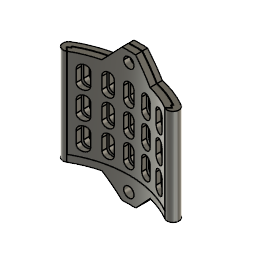
Mark 10 (Fusion) (Autodesk Fusion 360 design; units mm, degrees)
Autodesk Fusion 360 part; units mm, degrees
sketch "Base" plane through (0, 0, 0) normal (0, 0, 1) x (1, 0, 0) in component "Mark 10"
  circle A0 centre (0, 0) radius 57.15
  line L0 (0, 0) -> (0, 91.0821) construction
  line L1 (0, 0) -> (-28.575, 49.4934) construction
  line L2 (0, 0) -> (57.15, 0) construction
  circle A1 centre (-30.325, 52.5244) radius 3.5
  line L3 (-28.575, 49.4934) -> (-32.075, 55.5555) construction
  line L4 (-32.075, 55.5555) -> (-31.209, 56.0555) construction
  line L5 (-31.209, 56.0555) -> (-29.209, 52.5914)
  line L6 (-29.209, 52.5914) -> (-30.941, 51.5914)
  line L7 (-30.941, 51.5914) -> (-28.575, 49.4934)
  line L8 (0, 57.15) -> (0, 61.15) construction
  circle A2 centre (0, 0) radius 61.15
  line L9 (0, 57.15) -> (0, 64.15) construction
  circle A3 centre (0, 0) radius 64.15
  line L10 (28.575, 49.4934) -> (32.075, 55.5555) construction
  line L11 (32.075, 55.5555) -> (31.209, 56.0555) construction
  line L12 (31.209, 56.0555) -> (29.209, 52.5914)
  line L13 (30.941, 51.5914) -> (28.575, 49.4934)
  line L14 (29.209, 52.5914) -> (30.941, 51.5914)
  circle A4 centre (30.325, 52.5244) radius 3.5
  circle A5 centre (0, 0) radius 92.9081
  point P0 (-29.7049, 53.4504)
  point P1 (-29.209, 52.5914)
  point P2 (29.7049, 53.4504)
  point P3 (29.209, 52.5914)
  dimension "d1" = 114.3
  dimension "d2" = 120
  dimension "d3" = 7
  dimension "d4" = 1
  dimension "d5" = 4
  dimension "d6" = 2
  dimension "d8" = 4
  dimension "d9" = 7
  constraint coincident A0.centre L0.start
  constraint vertical L0
  constraint horizontal L2
  constraint coincident L1.end A1
  constraint coincident A1 L3.end
  constraint parallel L1 L3
  constraint perpendicular L3 L4
  constraint perpendicular L5 L6
  constraint perpendicular L4 L5
  constraint tangent A0 A1
  constraint coincident A0 L8.start
  constraint coincident L0 L8.start
  constraint parallel L0 L8
  constraint coincident L8.end A2
  constraint parallel L0 L9
  constraint coincident L9.end A3
  constraint coincident A2 P0
  constraint coincident L5 P0
  constraint coincident P1 L5.end
  constraint symmetric L0 L1.end L10.start
  constraint symmetric L0 A1 A4
  constraint symmetric L0 L3.end L10.end
  constraint symmetric L0 L4.end L11.end
  constraint symmetric L0 P1 P3
  constraint symmetric L0 L6.end L13.start
  constraint symmetric L0 P0 P2
  constraint concentric A2 A5
  measures "d1" diameter of A0
  measures "d2" angle of L1 L2
  measures "d3" diameter of A1
  measures "d4" distance of L3.end L4.end
  measures "d5" distance of L4.end P1
  measures "d6" distance of P1 L6.end
  measures "d8" distance of L8.start L8.end
  measures "d9" distance of L8.start L9.end
extrude "Extrude1" add sketch "Base" against normal blind 4 contours A2 L12 L13 L14 A4 | A0 A1 A2 A4 | A2 L12 L13 L14 A4 | A1 L5 L6 L7 A2 | A1 L5 L6 L7 A2 | A2 L12 A4 | A1 L5 A2 A3 L12 A4 | A2 L12 A4 | A1 L5 A2 | A1 L5 A2 picked at (17.8687, 55.5667) makes body 1 in component "Mark 10"
extrude "Extrude2" add sketch "Base" along normal blind 52 contours A2 L12 L13 L14 A4 | A1 L5 L6 L7 A2 | A2 L12 A4 | A1 L5 A2 A3 L12 A4 | A2 L12 A4 | A1 L5 A2 | A1 L5 A2 picked at (31.9687, 51.1565) picked at (-31.9687, 51.1565) bodies 1 in component "Mark 10"
ref_plane "WorkPlane1" through (0, 64.15, -0.6684) normal (0, 1, 0) x (-1, 0, 0) in component "Mark 10"
sketch "Screw Holes" plane through (0, 64.15, 0) normal (0, 1, 0) x (1, 0, 0) in component "Mark 10"
  line L0 (31.2051, 4) -> (-31.2051, 4)
  line L1 (0, 0) -> (0, 28) construction
  arc A0 through (-28.575, 4, -14.6566) (0, 4, -7) (28.575, 4, -14.6566) construction
  line L2 (0, 4) -> (0, 5.625) construction
  line L3 (0, 5.625) -> (0, 8.625) construction
  circle A1 centre (0, 8.625) radius 3
  line L4 (0, 8.625) -> (0, -24) construction
  line L5 (0, -24) -> (8, -24) construction
  line L6 (0, 4) -> (14, 4) construction
  line L7 (0, 11.625) -> (0, 14.625) construction
  line L8 (0, 14.625) -> (4, 14.625)
  line L9 (14, 4) -> (4, 14.625)
  line L10 (-14, 4) -> (-4, 14.625)
  line L11 (0, 14.625) -> (-4, 14.625)
  dimension "d16" = 1.625
  dimension "d17" = 3
  dimension "d18" = 32.625
  dimension "d19" = 3
  constraint coincident L1.start origin
  constraint perpendicular L0 L1
  constraint midpoint L0 L2.start
  constraint perpendicular L0 L2
  constraint parallel L1 L3
  constraint coincident L3.end A1.centre
  constraint coincident L2.end A1
  constraint parallel L3 L4
  constraint perpendicular L4 L5
  constraint coincident L0 L6.end
  constraint coincident A1 L7.start
  constraint coincident L1 L7.start
  constraint coincident L1 L7.end
  constraint perpendicular L1 L8
  constraint symmetric L1 L6.end L10.start
  constraint symmetric L1 L7.end L8.start
  constraint symmetric L1 L8.end L10.end
  measures "d16" distance of L2.start L2.end
  measures "d17" distance of L2.end L3.end
  measures "d18" distance of L3.end L4.end
  measures "d19" distance of L7.start L7.end
extrude "Extrude3" add sketch "Screw Holes" along normal blind -13 and the other way blind -2 bodies 1 in component "Mark 10"
ref_plane "WorkPlane2" through (4, 64.15, 24) normal (0, 0, 1) x (1, 0, 0) in component "Mark 10"
mirror "Mirror1" about plane through (4, 64.15, 24) normal (0, 0, 1) of "Extrude3" in component "Mark 10"
extrude "Extrude4" cut sketch "Base" along normal mid plane 150 contours A0 | A5 bodies 1 in component "Mark 10"
extrude "Extrude5" cut sketch "Base" along normal blind 70 contours A0 A1 A2 A4 picked at (17.8687, 55.5667) bodies 1 in component "Mark 10"
sketch "Base (2)" plane through (0, 0, 0) normal (0, 0, 1) x (-1, 0, 0) in component "Lid"
  line L0 (-28.575, -49.4934) -> (-30.941, -51.5914)
  line L1 (-30.941, -51.5914) -> (-29.209, -52.5914)
  line L2 (-29.209, -52.5914) -> (-29.7049, -53.4504)
  arc A0 (-29.7049, -53.4504) -> (29.7049, -53.4504) centre (0, 0) ccw
  line L3 (29.7049, -53.4504) -> (29.209, -52.5914)
  line L4 (29.209, -52.5914) -> (30.941, -51.5914)
  line L5 (30.941, -51.5914) -> (28.575, -49.4934)
  arc A1 (-28.575, -49.4934) -> (28.575, -49.4934) centre (0, 0) ccw
  line L6 (28.575, -49.4934) -> (28.4014, -49.5926) construction
  line L7 (30.941, -51.5914) -> (30.541, -51.5914) construction
  line L8 (28.4014, -49.5926) -> (30.541, -51.5914)
  circle A2 centre (0, 0) radius 59.9536
  arc A3 (-4, -64.0252) -> (4, -64.0252) centre (0, 0) ccw
  line L9 (0, -57.15) -> (0, -52.5675) construction
  line L10 (-28.4014, -49.5926) -> (-30.541, -51.5914)
  dimension "d31" = 0.2
  dimension "d32" = 0.4
  constraint coincident L5.end A1.end
  constraint coincident L4.end L5.start
  constraint horizontal L7
  constraint concentric A0 A2
  constraint coincident L7.end A2
  constraint midpoint A1 L9.start
  constraint vertical L9
  constraint symmetric L6.end L9 L10.start
  constraint symmetric L7.end L9 L10.end
  measures "d31" distance of L5.end L6.end
  measures "d32" distance of L4.end L7.end
extrude "Extrude1'" add sketch "Base (2)" along normal blind 52 separate body contours A1 L8 A2 L10 makes body 2 in component "Lid"
sketch "Hole Cover" plane through (0, 0, 52) normal (0, 0, 1) x (-1, 0, 0) in component "Lid"
  arc A0 (-30.541, -51.5914) -> (30.541, -51.5914) centre (0, 0) ccw
  line L0 (30.541, -51.5914) -> (28.4017, -49.593)
  arc A1 (-28.4017, -49.593) -> (28.4017, -49.593) centre (0, 0) ccw
  line L1 (-28.4017, -49.593) -> (-30.541, -51.5914)
  line L2 (29.209, -52.5914) -> (29.7049, -53.4504) construction
  line L3 (29.7049, -53.4504) -> (29.1066, -52.4141) construction
  line L4 (-28.575, -49.4934) -> (-30.941, -51.5914) construction
  line L5 (-30.941, -51.5914) -> (-29.209, -52.5914) construction
  line L6 (-29.209, -52.5914) -> (-29.7049, -53.4504) construction
  arc A2 (-29.7049, -53.4504) -> (29.7049, -53.4504) centre (0, 0) ccw construction
  line L7 (29.7049, -53.4504) -> (29.209, -52.5914) construction
  line L8 (29.209, -52.5914) -> (30.941, -51.5914) construction
  line L9 (30.941, -51.5914) -> (28.575, -49.4934) construction
  arc A3 (-28.575, -49.4934) -> (28.575, -49.4934) centre (0, 0) ccw construction
  line L10 (28.7992, -52.4816) -> (30.4306, -51.5397) construction
  line L11 (30.4306, -51.5397) -> (28.5374, -49.861) construction
  arc A4 (-28.5374, -49.861) -> (28.5374, -49.861) centre (0, 0) ccw construction
  line L12 (-28.5374, -49.861) -> (-30.4306, -51.5397) construction
  line L13 (-30.4306, -51.5397) -> (-28.7992, -52.4816) construction
  line L14 (-28.7992, -52.4816) -> (-29.2922, -53.3356) construction
  arc A5 (-29.2922, -53.3356) -> (29.2922, -53.3356) centre (0, 0) ccw
  line L15 (29.2922, -53.3356) -> (28.7992, -52.4816) construction
  line L16 (29.2922, -53.3356) -> (28.8439, -52.5591)
  line L17 (0, -60.85) -> (0, -66.5) construction
  line L18 (-29.2922, -53.3356) -> (-28.8439, -52.5591)
  dimension "d48" = -0.3
  constraint coincident L2.end L3.start
  constraint coincident A0 L3.end
  constraint parallel L2 L3
  constraint coincident L15 L16.end
  constraint coincident A0 L16.end
  constraint midpoint A5 L17.start
  constraint vertical L17
  constraint symmetric A5.end L17 L14.end
  constraint symmetric L16.end L17 L18.end
extrude "Extrude5'" add sketch "Hole Cover" against normal blind 2 contours A0 A5 L16 L18 bodies 2 in component "Lid"
sketch "Remover" plane through (0, 0, 52) normal (0, 0, 1) x (-1, 0, 0) in component "Lid"
  arc A0 (-30.541, -51.5914) -> (-28.8439, -52.5591) centre (0, 0) ccw
  line L0 (-28.8439, -52.5591) -> (-29.2922, -53.3356)
  arc A1 (-29.2922, -53.3356) -> (29.2922, -53.3356) centre (0, 0) ccw
  line L1 (29.2922, -53.3356) -> (28.8439, -52.5591)
  arc A2 (28.8439, -52.5591) -> (30.541, -51.5914) centre (0, 0) ccw
  line L2 (30.541, -51.5914) -> (28.4017, -49.593)
  arc A3 (-28.4017, -49.593) -> (28.4017, -49.593) centre (0, 0) ccw
  line L3 (-28.4017, -49.593) -> (-30.541, -51.5914)
  line L4 (39.8486, -52.3252) -> (29.1019, -42.286)
  arc A4 (-29.1019, -42.286) -> (29.1019, -42.286) centre (0, 0) ccw
  line L5 (-29.1019, -42.286) -> (-39.8486, -52.3252)
  arc A5 (-39.8486, -52.3252) -> (-36.7202, -54.5662) centre (0, 0) ccw
  line L6 (-36.7202, -54.5662) -> (-37.1695, -55.3443)
  arc A6 (-37.1695, -55.3443) -> (37.1695, -55.3443) centre (0, 0) ccw
  line L7 (37.1695, -55.3443) -> (36.7202, -54.5662)
  arc A7 (36.7202, -54.5662) -> (39.8486, -52.3252) centre (0, 0) ccw
  dimension "d51" = -5.8175
ref_plane "WorkPlane4" through (0, 60.85, 51.9755) normal (0, 1, 0) x (-1, 0, 0) in component "Lid"
sketch "Screw Hole" plane through (0, 60.85, 0) normal (0, 1, 0) x (1, 0, 0) in component "Lid"
  line L0 (14, -52) -> (4, -62.625)
  line L1 (4, -62.625) -> (-4, -62.625)
  line L2 (-4, -62.625) -> (-14, -52)
  spline S0 degree 3 poles (-3, -56.625) (-3, -56.2482) (-2.9247, -55.8464) (-2.6185, -55.1073) (-2.3876, -54.77) (-1.855, -54.2374) (-1.5177, -54.0065) (-0.7786, -53.7003) (-0.3768, -53.625) (0.3768, -53.625) (0.7786, -53.7003) (1.5177, -54.0065) (1.855, -54.2374) (2.3876, -54.77) (2.6185, -55.1073) (2.9247, -55.8464) (3, -56.2482) (3, -57.0018) (2.9247, -57.4036) (2.6185, -58.1427) (2.3876, -58.48) (1.855, -59.0126) (1.5177, -59.2435) (0.7786, -59.5497) (0.3768, -59.625) (-0.3768, -59.625) (-0.7786, -59.5497) (-1.5177, -59.2435) (-1.855, -59.0126) (-2.3876, -58.48) (-2.6185, -58.1427) (-2.9247, -57.4036) (-3, -57.0018) (-3, -56.625) knots 0 0 0 0 0.113025 0.113025 0.226051 0.226051 0.339076 0.339076 0.452102 0.452102 0.565127 0.565127 0.678153 0.678153 0.791178 0.791178 0.904204 0.904204 1.017229 1.017229 1.130255 1.130255 1.24328 1.24328 1.356306 1.356306 1.469331 1.469331 1.582357 1.582357 1.695382 1.695382 1.808407 1.808407 1.808407 1.808407
  line L3 (-29.2922, -52) -> (29.2922, -52)
extrude "Extrude6" add sketch "Screw Hole" against normal blind 7 bodies 2 in component "Lid"
extrude "Extrude7" cut sketch "Remover" along normal blind 14 bodies 2 in component "Lid"
ref_plane "WorkPlane1" through (0, 57.15, 36.0422) normal (0, -1, 0) x (-1, 0, 0)
ref_plane "WorkPlane2" through (0, 42.15, 36.0422) normal (0, -1, 0) x (-1, 0, 0)
sketch "Holes" plane through (0, 42.15, 0) normal (0, -1, 0) x (-1, 0, 0)
  line L0 (28.575, 0) -> (28.575, -52)
  line L1 (-28.575, 0) -> (-28.575, -52)
  line L2 (-28.4017, 0) -> (28.4017, 0)
  circle A0 centre (22, -6) radius 3
  circle A1 centre (22, -13) radius 3
  line L3 (19, -5.9862) -> (19, -13)
  line L4 (24.9846, -13.3033) -> (25, -6.0063)
  line L5 (13.9846, -13.3033) -> (14, -6.0063)
  line L6 (8, -5.9862) -> (8, -13)
  circle A2 centre (11, -6) radius 3
  circle A3 centre (11, -13) radius 3
  line L7 (2.9846, -13.3033) -> (3, -6.0063)
  line L8 (-3, -5.9862) -> (-3, -13)
  circle A4 centre (0, -6) radius 3
  circle A5 centre (0, -13) radius 3
  line L9 (-8.0154, -13.3033) -> (-8, -6.0063)
  line L10 (-14, -5.9862) -> (-14, -13)
  circle A6 centre (-11, -6) radius 3
  circle A7 centre (-11, -13) radius 3
  line L11 (-19.0154, -13.3033) -> (-19, -6.0063)
  line L12 (-25, -5.9862) -> (-25, -13)
  circle A8 centre (-22, -6) radius 3
  circle A9 centre (-22, -13) radius 3
  line L13 (24.9846, -28.8033) -> (25, -21.5063)
  line L14 (19, -21.4862) -> (19, -28.5)
  circle A10 centre (22, -21.5) radius 3
  circle A11 centre (22, -28.5) radius 3
  line L15 (13.9846, -28.8033) -> (14, -21.5063)
  line L16 (8, -21.4862) -> (8, -28.5)
  circle A12 centre (11, -21.5) radius 3
  circle A13 centre (11, -28.5) radius 3
  line L17 (2.9846, -28.8033) -> (3, -21.5063)
  line L18 (-3, -21.4862) -> (-3, -28.5)
  circle A14 centre (0, -21.5) radius 3
  circle A15 centre (0, -28.5) radius 3
  line L19 (-8.0154, -28.8033) -> (-8, -21.5063)
  line L20 (-14, -21.4862) -> (-14, -28.5)
  circle A16 centre (-11, -21.5) radius 3
  circle A17 centre (-11, -28.5) radius 3
  line L21 (-19.0154, -28.8033) -> (-19, -21.5063)
  line L22 (-25, -21.4862) -> (-25, -28.5)
  circle A18 centre (-22, -21.5) radius 3
  circle A19 centre (-22, -28.5) radius 3
  line L23 (24.9846, -44.3033) -> (25, -37.0063)
  line L24 (19, -36.9862) -> (19, -44)
  circle A20 centre (22, -37) radius 3
  circle A21 centre (22, -44) radius 3
  line L25 (13.9846, -44.3033) -> (14, -37.0063)
  line L26 (8, -36.9862) -> (8, -44)
  circle A22 centre (11, -37) radius 3
  circle A23 centre (11, -44) radius 3
  line L27 (2.9846, -44.3033) -> (3, -37.0063)
  line L28 (-3, -36.9862) -> (-3, -44)
  circle A24 centre (0, -37) radius 3
  circle A25 centre (0, -44) radius 3
  line L29 (-8.0154, -44.3033) -> (-8, -37.0063)
  line L30 (-14, -36.9862) -> (-14, -44)
  circle A26 centre (-11, -37) radius 3
  circle A27 centre (-11, -44) radius 3
  line L31 (-19.0154, -44.3033) -> (-19, -37.0063)
  line L32 (-25, -36.9862) -> (-25, -44)
  circle A28 centre (-22, -37) radius 3
  circle A29 centre (-22, -44) radius 3
  dimension "d59" = 6
  dimension "d72" = 6
  dimension "d75" = -44
  dimension "d76" = -31
  constraint coincident A0 L3.start
  constraint coincident A1 L3.end
  constraint tangent A1 L3
  constraint coincident A1 L4.start
  constraint coincident A0 L4.end
  constraint tangent A0 L4
  measures "d59" diameter of A0
  measures "d72" diameter of A1
extrude "Extrude8" cut sketch "Holes" against normal blind 58 bodies 1 in component "Mark 10"
extrude "Extrude9" cut sketch "Holes" against normal blind 58 bodies 2 in component "Lid"
sketch "Screw dia check" plane through (0, 121.7984, 0) normal (0, 1, 0) x (-1, 0, 0)
  ellipse E0 centre (45.9857, 66.482) end of major axis (44.3189, 66.3475) minor radius 1.6722 (46.0443, 64.8108) -> (46.1957, 64.823) ccw
  arc A0 (46.1957, 64.823) -> (47.2938, 65.272) centre (46.1957, 66.3903) ccw
  ellipse E1 centre (46.4026, 66.4799) end of major axis (45.238, 65.5327) minor radius 1.5011 (47.2938, 65.272) -> (47.4035, 65.3612) ccw
  arc A1 (47.4035, 65.3612) -> (46.0443, 64.8108) centre (46.1957, 66.3903) ccw
  circle A2 centre (46.1957, 66.3903) radius 2.1336
  dimension "d81" = 4.2672
  measures "d81" diameter of A2
sketch "Placement distances" plane through (0, 0, 0) normal (0, 1, 0) x (1, 0, 0)
  spline S0 degree 3 poles (-3, -56.625) (-3, -56.4159) (-2.9781, -56.2074) (-2.8902, -55.7925) (-2.8231, -55.5876) (-2.5701, -55.0265) (-2.3339, -54.698) (-1.7581, -54.1639) (-1.4282, -53.9588) (-0.6946, -53.6792) (-0.296, -53.6129) (0.4893, -53.6402) (0.8684, -53.7277) (1.5871, -54.0477) (1.9172, -54.2829) (2.454, -54.857) (2.6602, -55.1858) (2.9416, -55.9148) (3.0097, -56.3096) (2.9885, -57.0912) (2.904, -57.4705) (2.5915, -58.1876) (2.3621, -58.5166) (1.798, -59.057) (1.4723, -59.2669) (0.7476, -59.5573) (0.3537, -59.6304) (-0.4273, -59.6192) (-0.8069, -59.5399) (-1.5274, -59.2374) (-1.8594, -59.0125) (-2.4068, -58.4564) (-2.6209, -58.1343) (-2.9213, -57.4145) (-3, -57.0218) (-3, -56.625) knots -1.891021 -1.891021 -1.891021 -1.891021 -1.828288 -1.828288 -1.763792 -1.763792 -1.643578 -1.643578 -1.528089 -1.528089 -1.408024 -1.408024 -1.29237 -1.29237 -1.171941 -1.171941 -1.056515 -1.056515 -0.937477 -0.937477 -0.821954 -0.821954 -0.702762 -0.702762 -0.587532 -0.587532 -0.468501 -0.468501 -0.353205 -0.353205 -0.23403 -0.23403 -0.119026 -0.119026 0 0 0 0
  line L0 (-17.9711, -42.2512) -> (17.0289, -42.2512)
  line L1 (17.0289, -7.2512) -> (-17.9711, -7.2512)
  spline S1 degree 3 poles (3, 8.625) (3, 8.2482) (2.9247, 7.8464) (2.6185, 7.1073) (2.3876, 6.77) (1.855, 6.2374) (1.5177, 6.0065) (0.7786, 5.7003) (0.3768, 5.625) (-0.3768, 5.625) (-0.7786, 5.7003) (-1.5177, 6.0065) (-1.855, 6.2374) (-2.3876, 6.77) (-2.6185, 7.1073) (-2.9247, 7.8464) (-3, 8.2482) (-3, 9.0018) (-2.9247, 9.4036) (-2.6185, 10.1427) (-2.3876, 10.48) (-1.855, 11.0126) (-1.5177, 11.2435) (-0.7786, 11.5497) (-0.3768, 11.625) (0.3768, 11.625) (0.7786, 11.5497) (1.5177, 11.2435) (1.855, 11.0126) (2.3876, 10.48) (2.6185, 10.1427) (2.9247, 9.4036) (3, 9.0018) (3, 8.625) knots 0 0 0 0 0.113028 0.113028 0.226057 0.226057 0.339085 0.339085 0.452113 0.452113 0.565141 0.565141 0.67817 0.67817 0.791198 0.791198 0.904226 0.904226 1.017255 1.017255 1.130283 1.130283 1.243311 1.243311 1.356339 1.356339 1.469368 1.469368 1.582396 1.582396 1.695424 1.695424 1.808453 1.808453 1.808453 1.808453
  line L2 (-3, -56.625) -> (3, -56.625) construction
  line L3 (0, -56.625) -> (0, -25) construction
  line L4 (3, 8.625) -> (-3, 8.625) construction
  spline S2 degree 3 poles (0, -59.625) (0.0344, -59.625) (0.0689, -59.6244) (0.4886, -59.6099) (0.8676, -59.5225) (1.5864, -59.2027) (1.9166, -58.9675) (2.4536, -58.3936) (2.6599, -58.0647) (2.9415, -57.3357) (3.0096, -56.9408) (2.9885, -56.1592) (2.9042, -55.78) (2.5918, -55.0628) (2.3624, -54.7338) (1.7984, -54.1933) (1.4727, -53.9833) (0.7612, -53.6981) (0.3823, -53.625) (0, -53.625) knots -1.418404 -1.418404 -1.418404 -1.418404 -1.408059 -1.408059 -1.292417 -1.292417 -1.171987 -1.171987 -1.05655 -1.05655 -0.937499 -0.937499 -0.821985 -0.821985 -0.702798 -0.702798 -0.587557 -0.587557 -0.472792 -0.472792 -0.472792 -0.472792
  point P0 (0, -42.2512)
  dimension "d82" = 14.3738
  dimension "d83" = 17.2512
  dimension "d84" = 17.7488
  dimension "d85" = 15.8762
  dimension "d86" = 65.25
  dimension "d87" = 31.625
  dimension "d88" = 33.625
  dimension "d90" = 6
  constraint coincident S0.start S0.end
  constraint coincident S0 L2.end
  constraint horizontal L2
  constraint midpoint L2 L3.start
  constraint perpendicular L2 L3
  constraint coincident L3 P0
  constraint coincident L0 P0
  constraint coincident S1.start S1.end
  constraint coincident S1 L4.end
  constraint horizontal L4
  measures "d82" distance of L3.start P0
  measures "d83" distance of L3.end P0
  measures "d84" distance of L1 L3.end
  measures "d85" distance of L1 L4
  measures "d86" distance of L3.start L4
  measures "d87" distance of L3.start L3.end
  measures "d88" distance of L3.end L4
  measures "d90" distance of S2.start S2.end
extrude "Extrude7'" [suppressed] in component "Mark 10"
extrude "Extrude8'" [no effect] in component "Lid"
emboss "Emboss1" [suppressed] in component "Lid"
component "Mark 10" placed x (1, 0, 0) y (0, 1, 0) z (0, 0, 1) at (0, 0, 0)
component "Lid" placed x (1, 0, 0) y (0, 1, 0) z (0, 0, 1) at (0, 0, 0)
equation "d2 = 90 deg + 30 deg"
equation "d16 = 1.5 mm + 0.125 mm"
